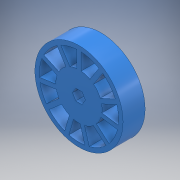
# Autodesk Inventor part: RobotArm Wheel
Saved by Autodesk Inventor 2018.2 (Build 222227000, 227)
## iProperties
Created: 2018-01-13
Part Number: RobotArm Wheel
Material: Generic
Document SubType Name: Modeling
Designer: lopez.xavier
Density: 1 g/cm^3
Appearance: Cyan
Author: lopez.xavier
Autodesk Inventor part; units mm, degrees
ref_plane "YZ Plane" through (0, 0, 0) normal (1, 0, 0) x (0, 1, 0)
ref_plane "XZ Plane" through (0, 0, 0) normal (0, 1, 0) x (-1, 0, 0)
ref_plane "XY Plane" through (0, 0, 0) normal (0, 0, 1) x (1, 0, 0)
sketch "Sketch1" plane through (0, 0, 0) normal (0, 0, 1) x (1, 0, 0)
  circle A0 centre (0, 0) radius 50.8
  circle A1 centre (0, 0) radius 45.72
  circle A2 centre (0, 0) radius 26.67
  circle A3 centre (0, 0) radius 19.05
  circle A4 centre (0, 0) radius 11.43
  line L0 (3.6662, 6.35) -> (7.3323, 0)
  line L1 (7.3323, 0) -> (3.6662, -6.35)
  line L2 (3.6662, -6.35) -> (-3.6662, -6.35)
  line L3 (-3.6662, -6.35) -> (-7.3323, 0)
  line L4 (-7.3323, 0) -> (-3.6662, 6.35)
  line L5 (-3.6662, 6.35) -> (3.6662, 6.35)
  line L6 (0, 0) -> (0, 58.0354)
  line L7 (-2.54, 26.5488) -> (-2.54, 45.6494)
  line L8 (2.54, 26.5488) -> (2.54, 45.6494)
  line L9 (12.7, 23.4521) -> (23.014, 39.5054)
  line L10 (16.9172, 20.6179) -> (27.2549, 36.7081)
  line L11 (24.5372, 10.4506) -> (41.8671, 18.3702)
  line L12 (43.6505, 13.5998) -> (26.0816, 5.571)
  line L13 (26.4637, -3.3108) -> (45.3226, -6.0149)
  line L14 (25.3511, -8.2832) -> (44.3743, -11.0109)
  line L15 (20.2711, -17.3312) -> (34.6746, -29.7992)
  line L16 (16.6011, -20.8733) -> (31.1496, -33.4667)
  line L17 (6.4411, -25.8805) -> (11.8225, -44.165)
  line L18 (1.3677, -26.6349) -> (6.8336, -45.2064)
  line L19 (-6.2201, -25.9345) -> (-11.577, -44.23)
  line L20 (-11.0296, -24.2824) -> (-16.4141, -42.672)
  line L21 (-19.9196, -17.7341) -> (-34.3062, -30.2225)
  line L22 (-22.9299, -13.6202) -> (-37.4507, -26.2252)
  line L23 (-25.9863, -6.0002) -> (-44.8776, -8.7359)
  line L24 (-26.6526, -0.9637) -> (-45.5698, -3.7032)
  line L25 (-25.2585, 8.5613) -> (-42.6471, 16.4785)
  line L26 (-23.177, 13.1954) -> (-40.5558, 21.108)
  line L27 (-14.9508, 22.0854) -> (-25.2719, 38.1005)
  line L28 (-10.4794, 24.5249) -> (-20.8849, 40.6711)
  dimension "d2" = 19.05
  dimension "d0" = 101.6
  dimension "d1" = 5.08
  dimension "d3" = 7.62
  dimension "d4" = 22.86
  dimension "d5" = 12.7
  dimension "d6" = 5.08
  dimension "d7" = 2.54
  dimension "d8" = 5.08
  dimension "d9" = 32.72
  dimension "d10" = 10.16
  dimension "d11" = 32.72
  dimension "d12" = 5.08
  dimension "d13" = 7.62
  dimension "d14" = 5.08
  dimension "d15" = 32.72
  dimension "d16" = 8.89
  dimension "d17" = 32.72
  dimension "d18" = 5.08
  dimension "d19" = 5.08
  dimension "d20" = 32.72
  dimension "d21" = 10.16
  dimension "d22" = 5.08
  dimension "d23" = 5.08
  dimension "d24" = 32.72
  dimension "d25" = 7.62
  dimension "d26" = 5.08
  dimension "d27" = 32.72
  dimension "d28" = 8.89
  dimension "d29" = 5.08
  dimension "d30" = 32.72
  dimension "d31" = 7.62
  dimension "d32" = 5.08
  dimension "d33" = 32.72
  dimension "d34" = 9.525
  dimension "d35" = 5.08
  dimension "d36" = 32.72
  dimension "d37" = 8.89
  constraints: 58 end point, 10 parallel, 6 coincident, 3 centre point, 3 vertical, 1 perpendicular, 61 other
  measures "d0" diameter of A0
  measures "d4" diameter of A4
  measures "d5" distance between parallel lines of L2 L5
  measures "d6" distance between parallel lines of L8 L7
  measures "d7" distance between parallel lines of L6 L7
  measures "d8" distance between parallel lines of L10 L9
  measures "d9" angle of L8 L9
  measures "d10" horizontal distance of L8.start L9.start
  measures "d11" angle of L10 L11
  measures "d12" distance between parallel lines of L11 L12
  measures "d13" horizontal distance of L11.start L10.start
  measures "d14" distance between parallel lines of L13 L14
  measures "d15" angle of L12 L13
  measures "d16" distance of L13.start L12.end
  measures "d17" angle of L14 L15
  measures "d18" horizontal distance of L14.start L15.start
  measures "d19" distance between parallel lines of L15 L16
  measures "d20" angle of L16 L17
  measures "d21" horizontal distance of L16.start L17.start
  measures "d22" distance between parallel lines of L17 L18
  measures "d23" distance between parallel lines of L20 L19
  measures "d24" angle of L18 L19
  measures "d25" distance of L18.start L19.start
  measures "d26" distance between parallel lines of L22 L21
  measures "d27" angle of L20 L21
  measures "d28" horizontal distance of L20.start L21.start
  measures "d29" distance between parallel lines of L23 L24
  measures "d30" angle of L22 L23
  measures "d31" vertical distance of L22.start L23.start
  measures "d32" distance between parallel lines of L26 L25
  measures "d33" angle of L24 L25
  measures "d34" vertical distance of L24.start L25.start
  measures "d35" distance between parallel lines of L28 L27
  measures "d36" angle of L26 L27
  measures "d37" vertical distance of L26.start L27.start
extrude "Extrusion3" add sketch "Sketch1" along normal blind 25.4 contours A1 L8 A2 L6 | L6 A2 L7 A1 | A0 | A2 | A4 | A1 L10 A2 L9 | L28 A2 L27 A1 | A1 L12 A2 L11 | L26 A2 L25 A1 | L24 A2 L23 A1 | A1 L14 A2 L13 | L22 A2 L21 A1 | A1 L16 A2 L15 | L20 A2 L19 A1 | A1 L18 A2 L17
sketch "Sketch3" plane through (0, 0, 25.4) normal (0, 0, 1) x (1, 0, 0)
  circle A0 centre (0, 0) radius 11.43 projected
  circle A1 centre (0, 0) radius 19.05 projected
extrude "Extrusion4" add sketch "Sketch3" against normal blind 2.54
sketch "Sketch4" plane through (0, 0, 22.86) normal (0, 0, -1) x (-1, 0, 0)
  circle A0 centre (0, 0) radius 11.43 projected
  line L0 (-10.4724, 4.5798) -> (-17.0961, 8.404)
  circle A1 centre (0, 0) radius 19.05 projected
  line L1 (-9.2024, 6.7795) -> (-15.8261, 10.6037)
  line L2 (-7.3323, 0) -> (-3.6662, 6.35) projected
  line L3 (-3.6662, 6.35) -> (-7.3323, 0) projected
  line L4 (-3.6662, 6.35) -> (-14.3563, 12.5219)
  line L5 (3.6662, 6.35) -> (-3.6662, 6.35) projected
  line L6 (-3.6662, 6.35) -> (3.6662, 6.35) projected
  line L7 (-1.27, -11.3592) -> (-1.27, -19.0076)
  line L8 (1.27, -11.3592) -> (1.27, -19.0076)
  line L9 (-3.6662, -6.35) -> (3.6662, -6.35) projected
  line L10 (-3.6662, -6.35) -> (-14.3563, -12.5219)
  line L11 (3.6662, -6.35) -> (14.3563, -12.5219)
  line L12 (3.6662, 6.35) -> (14.3563, 12.5219)
  line L13 (-3.6662, -6.35) -> (-7.3323, 0) projected
  line L14 (3.6662, 6.35) -> (7.3323, 0) projected
  line L15 (7.3323, 0) -> (3.6662, -6.35) projected
  line L16 (10.4724, -4.5798) -> (17.0961, -8.404)
  line L17 (9.2024, -6.7795) -> (15.8261, -10.6037)
  line L18 (-10.4724, -4.5798) -> (-17.0961, -8.404)
  line L19 (-9.2024, -6.7795) -> (-15.8261, -10.6037)
  line L20 (9.2024, 6.7795) -> (15.8261, 10.6037)
  line L21 (10.4724, 4.5798) -> (17.0961, 8.404)
  line L22 (-3.6662, 6.35) -> (-3.6662, 18.6939)
  line L23 (3.6662, -6.35) -> (3.6662, -18.6939)
  line L24 (3.6662, -6.35) -> (-3.6662, -6.35) projected
  line L25 (-1.27, 11.3592) -> (-1.27, 19.0076)
  line L26 (1.27, 11.3592) -> (1.27, 19.0076)
  dimension "d57" = 2.54
  dimension "d62" = 2.54
  dimension "d64" = 2.54
  dimension "d66" = 2.54
  dimension "d68" = 2.54
  dimension "d72" = 2.3962
  dimension "d73" = 2.3962
  dimension "d74" = 2.3962
  dimension "d75" = 2.3962
  dimension "d76" = 2.3962
  dimension "d77" = 2.3962
  dimension "d78" = 2.54
  constraints: 36 end point, 11 perpendicular, 6 parallel, 32 other
  measures "d57" distance between parallel lines of L0 L1
  measures "d62" distance between parallel lines of L7 L8
  measures "d64" distance between parallel lines of L16 L17
  measures "d66" distance between parallel lines of L18 L19
  measures "d68" distance between parallel lines of L20 L21
  measures "d72" distance between parallel lines of L1 L4
  measures "d73" distance between parallel lines of L20 L12
  measures "d74" distance between parallel lines of L11 L17
  measures "d75" distance between parallel lines of L8 L23
  measures "d76" distance between parallel lines of L19 L10
  measures "d77" distance between parallel lines of L22 L25
  measures "d78" distance between parallel lines of L25 L26
extrude "Extrusion5" add sketch "Sketch4" along normal blind 16.51 contours A0 L20 A1 L21 | L16 A1 L17 A0 | A0 L25 A1 L26 | L8 A1 L7 A0 | A0 L0 A1 L1 | L19 A1 L18 A0
equation "\"d11\" = d9"
equation "\"d15\" = d11"
equation "\"d17\" = d9"
equation "\"d20\" = d9"
equation "\"d24\" = d9"
equation "\"d27\" = d9"
equation "\"d30\" = d9"
equation "\"d33\" = d9"
equation "\"d36\" = d9"
body "Solid2"
